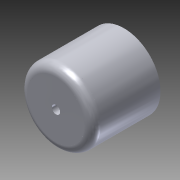
# Autodesk Inventor part: Long Cap .125 Hole
Saved by Autodesk Inventor 2013 (Build 170138000, 138)
## iProperties
Created: 2013-06-27
Part Number: Long Cap .125 Hole
Material: PVC-Piping
Document SubType Name: Modeling
Designer: Kyle
Density: 1 g/cm^3
Author: Kyle
Autodesk Inventor part; units mm, degrees
ref_plane "YZ Plane" through (0, 0, 0) normal (1, 0, 0) x (0, 1, 0)
ref_plane "XZ Plane" through (0, 0, 0) normal (0, 1, 0) x (-1, 0, 0)
ref_plane "XY Plane" through (0, 0, 0) normal (0, 0, 1) x (1, 0, 0)
sketch "Sketch1" plane through (0, 0, 0) normal (0, 0, 1) x (1, 0, 0)
  circle A0 centre (0, 0) radius 13.97
  circle A1 centre (0, 0) radius 10.795
  dimension "d0" = 27.94
  dimension "d2" = 21.59
  constraints: 2 centre point, 2 coincident
  measures "d0" diameter of A0
  measures "d2" diameter of A1
extrude "Extrusion1" add sketch "Sketch1" along normal blind 13.335
sketch "Sketch2" plane through (0, 0, 13.335) normal (0, 0, 1) x (1, 0, 0)
  circle A0 centre (0, 0) radius 13.97 projected
extrude "Extrusion2" add sketch "Sketch2" along normal blind 3.175
fillet "Fillet1" radius 3.175 1 edges at (-13.97, 0, 16.51)
sketch "Sketch3" plane through (0, 0, 0) normal (0, 0, -1) x (-1, 0, 0)
  circle A0 centre (0, 0) radius 10.795 projected
  circle A1 centre (0, 0) radius 13.97 projected
extrude "Extrusion3" add sketch "Sketch3" along normal blind 1.27
sketch "Sketch4" plane through (0, 0, -1.27) normal (0, 0, -1) x (-1, 0, 0)
  circle A0 centre (0, 0) radius 10.795 projected
  circle A1 centre (0, 0) radius 13.97 projected
extrude "Extrusion4" cut sketch "Sketch4" along normal blind 5.715
sketch "Sketch5" plane through (0, 0, -1.27) normal (0, 0, -1) x (-1, 0, 0)
  circle A0 centre (0, 0) radius 10.795 projected
  circle A1 centre (0, 0) radius 13.97 projected
extrude "Extrusion5" add sketch "Sketch5" along normal blind 8.255
sketch "Sketch6" plane through (0, 0, 16.51) normal (0, 0, 1) x (1, 0, 0)
  circle A0 centre (0, 0) radius 10.795 projected
  circle A1 centre (0, 0) radius 1.5875
  dimension "d14" = 3.175
  constraints: 1 centre point, 1 coincident
  measures "d14" diameter of A1
extrude "Extrusion6" cut sketch "Sketch6" against normal blind 25.4 contours A1
body "Solid1"
